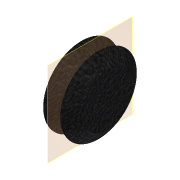
# Autodesk Inventor part: Neje_Rolls
Saved by Autodesk Inventor 2019.4 (Build 234330000, 330)
## iProperties
Created: 2021-04-08
Part Number: Neje_Rolls
Material: Generic
Document SubType Name: Modeling
Designer: diederichbenedict
Density: 1 g/cm^3
Appearance: Black Cast
Author: diederichbenedict
Autodesk Inventor part; units mm, degrees
ref_plane "YZ Plane" through (0, 0, 0) normal (1, 0, 0) x (0, 1, 0)
ref_plane "XZ Plane" through (0, 0, 0) normal (0, 1, 0) x (-1, 0, 0)
ref_plane "XY Plane" through (0, 0, 0) normal (0, 0, 1) x (1, 0, 0)
sketch "Sketch1" plane through (0, 0, 0) normal (0, 0, 1) x (1, 0, 0)
  line L0 (0, 0) -> (0, 8.4)
  line L1 (0, 0) -> (-11, 0)
  line L2 (-11, 0) -> (-11, 8.4)
  line L3 (-8.25, 0) -> (-8.25, 12.4)
  line L4 (-11, 8.4) -> (-8.25, 12.4)
  line L5 (-8.25, 12.4) -> (-5.5, 8.4)
  line L6 (-5.5, 8.4) -> (-5.5, 0)
  line L7 (0, 8.4) -> (-2.75, 12.4)
  line L8 (-2.75, 12.4) -> (-5.5, 8.4)
  dimension "d0" = 11
  dimension "d1" = 12.4
  dimension "d2" = 8.4
  dimension "d3" = 2.75
  dimension "d4" = 5.5
  dimension "d5" = 2.75
  constraints: 18 end point, 2 perpendicular, 2 vertical, 1 horizontal, 1 midpoint, 1 point on line
  measures "d0" distance of L0.start L1.end
  measures "d1" distance of L3.start L3.end
  measures "d2" distance of L0.start L0.end
  measures "d3" distance between parallel lines of L3 L2
  measures "d4" distance between parallel lines of L6 L2
  measures "d5" distance from line of L7.end L0
revolve "Revolution1" add sketch "Sketch1" angle 360 about axis through (0, 0, 0) along (-1, 0, 0)
ref_plane "Work Plane1" through (-5.5, 0, 0) normal (1, 0, 0) x (0, 0, -1)
body "Solid1"
